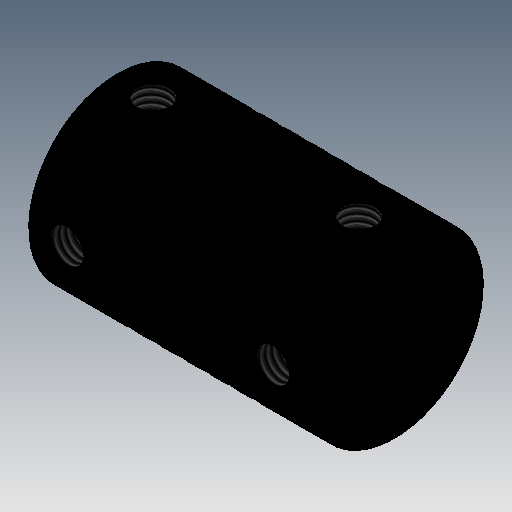
# Autodesk Inventor part: MCJN14-4-4_body
Saved by Autodesk Inventor 2019.4 (Build 234330000, 330)
## iProperties
Category: PARTsolutions
Company: MISUMI
Created: 2019-06-16
Part Number: MCJN14-4-4_body
Material: 一般
Catalog Web Link: www.cadenas.de
Description: MCJN_body-Couplings - Resin Type
Vendor: MISUMI
Document SubType Name: Modeling
Designer: psadmin
Manufacturer: MISUMI
Mass: 2.07781 g
Surface Area: 25.8504 cm^2
Volume: 2.07781 cm^3
Density: 1 g/cm^3
Appearance: PSOLRGB-0-0-0
PSOL_IDENT_0: {$CADENAS_DATA\23d-libs\misumi\metric\50_couplings\mcjn.prj},175 {VTYP=3D},{NB=MCJN14-4-4_body},{LIN
PSOL_IDENT_1: A=MCJN14-4-4},{NN=MCJN_body},{DATE=30.03.2018 07:24:16},{GEOMDATE=10.09.2008 06:56:00},{VERSION=},{L
PSOL_IDENT_2: INEID=20},{WBVAR=DD1,DD2},{WBNUMERIC=}  {NB=MCJN14-4-4_body},{LINA=MCJN14-4-4},{KT=DUMMY},{PN=MCJN14
PSOL_IDENT_3: -4-4},{MAT=Glass Fiber Reinforced PBT Resin},{AC=Set Screw},{TYPE=MCJN},{NO=14},{DD1=4},{DD1ALG1='4'
PSOL_IDENT_4: ,'4'},{DD1ALG2=4},{DD2=4},{DD2ALG1='2.5','2.5','3','3','3.2','3.2','4','4'},{DD2ALG2=4},{D=13.5},{DI
PSOL_IDENT_5: A=13.500},{L=21},{L1=21},{LL1=21},{LL11=21.000},{LL=5.3},{F=2.7},{M=M3X5},{T=0.2},{DL=4},{DR=4},{TSI
PSOL_IDENT_6: MD=3.000},{TSIMIN=2.459},{DIA1=2.8400},{L11=0.950},{L2=3.780},{L3=1.900},{TSS=3.000},{LSS=5.000}
NN: MCJN_body
NT: Couplings - Resin Type
NB: MCJN14-4-4_body
NBSYN: $TYPE.$NO.-$DD1.-$DD2._body
LINA: MCJN14-4-4
PN: MCJN14-4-4
MAT: Glass Fiber Reinforced PBT Resin
AC: Set Screw
NO: 14
DD1: 4
DD2: 4
D: 13.5
L: 21
LL: 5.3
F: 2.7
M: M3X5
T: 0.2
SUPPLIER: MISUMI
ARTICLENO: MCJN14-4-4_body
BOMINFO: MCJN14-4-4
CREATOR: CADENAS GmbH
Title: MCJN14-4-4
Author: Cadenas PARTsolutions
Comments: Couplings - Resin Type
Autodesk Inventor part; units mm, degrees
sketch "Sketch_1" plane through (0, 0, 0) normal (0, 0, 1) x (1, 0, 0)
  line L0 (21, 0) -> (0, 0)
  line L1 (0, 0) -> (0, 6.75)
  line L2 (0, 6.75) -> (21, 6.75)
  line L3 (21, 6.75) -> (21, 0)
  line L4 (21, 0) -> (0, 0)
  constraints: 10 end point
revolve "Revolution1" add sketch "Sketch_1" angle 360 about axis through (21, 0, 0) along (1, 0, 0)
sketch "Sketch_2" plane through (0, 0, 0) normal (0, 0, 1) x (1, 0, 0)
  line L0 (15.7, 0) -> (0, 0)
  line L1 (0, 0) -> (0, 2)
  line L2 (0, 2) -> (15.7, 2)
  line L3 (15.7, 2) -> (15.7, 0)
  line L4 (15.7, 0) -> (0, 0)
  constraints: 10 end point
revolve "Revolution2" cut sketch "Sketch_2" angle 360 about axis through (15.7, 0, 0) along (1, 0, 0)
sketch "Sketch3" plane through (21, 0, 0) normal (1, 0, 0) x (0, 0, -1)
  point P0 (0, 0)
hole "Hole1" at (21, 0, 0) direction (-1, 0, 0) diameter 4 depth 5.3
sketch "Sketch_4" plane through (0, 0, 0) normal (0, 0, 1) x (1, 0, 0)
  arc A0 (5.3, 1.9) -> (6.25, 1.9) centre (5.775, 1.9) ccw
  line L0 (6.25, 1.9) -> (6.25, 6.75)
  line L1 (6.25, 6.75) -> (9.125, 6.75)
  line L2 (9.125, 6.75) -> (9.125, 1.9)
  arc A1 (9.125, 1.9) -> (10.075, 1.9) centre (9.6, 1.9) ccw
  line L3 (10.075, 1.9) -> (10.075, 6.75)
  line L4 (10.075, 6.75) -> (12.85, 6.75)
  line L5 (12.85, 6.75) -> (12.85, 1.9)
  arc A2 (12.85, 1.9) -> (13.8, 1.9) centre (13.325, 1.9) ccw
  line L6 (13.8, 1.9) -> (13.8, 8.1)
  line L7 (13.8, 8.1) -> (5.3, 8.1)
  line L8 (5.3, 8.1) -> (5.3, 1.9)
  constraints: 18 end point, 6 point on circle, 3 centre point
extrude "Extrusion1" cut sketch "Sketch_4" along normal mid plane 13.5
sketch "Sketch_5" plane through (0, 0, 0) normal (0, 0, 1) x (1, 0, 0)
  line L0 (5.3, -1.9) -> (5.3, -8.1)
  line L1 (5.3, -8.1) -> (13.8, -8.1)
  line L2 (13.8, -8.1) -> (13.8, -1.9)
  arc A0 (13.8, -1.9) -> (12.85, -1.9) centre (13.325, -1.9) ccw
  line L3 (12.85, -1.9) -> (12.85, -6.75)
  line L4 (12.85, -6.75) -> (10.075, -6.75)
  line L5 (10.075, -6.75) -> (10.075, -1.9)
  arc A1 (10.075, -1.9) -> (9.125, -1.9) centre (9.6, -1.9) ccw
  line L6 (9.125, -1.9) -> (9.125, -6.75)
  line L7 (9.125, -6.75) -> (6.25, -6.75)
  line L8 (6.25, -6.75) -> (6.25, -1.9)
  arc A2 (6.25, -1.9) -> (5.3, -1.9) centre (5.775, -1.9) ccw
  constraints: 18 end point, 6 point on circle, 3 centre point
extrude "Extrusion2" cut sketch "Sketch_5" along normal mid plane 13.5
sketch "Sketch_6" plane through (0, 0, 0) normal (0, 1, 0) x (-1, 0, 0)
  arc A0 (-7.2, -1.9) -> (-8.15, -1.9) centre (-7.675, -1.9) ccw
  line L0 (-8.15, -1.9) -> (-8.15, -6.75)
  line L1 (-8.15, -6.75) -> (-11.025, -6.75)
  line L2 (-11.025, -6.75) -> (-11.025, -1.9)
  arc A1 (-11.025, -1.9) -> (-11.975, -1.9) centre (-11.5, -1.9) ccw
  line L3 (-11.975, -1.9) -> (-11.975, -6.75)
  line L4 (-11.975, -6.75) -> (-14.75, -6.75)
  line L5 (-14.75, -6.75) -> (-14.75, -1.9)
  arc A2 (-14.75, -1.9) -> (-15.7, -1.9) centre (-15.225, -1.9) ccw
  line L6 (-15.7, -1.9) -> (-15.7, -8.1)
  line L7 (-15.7, -8.1) -> (-7.2, -8.1)
  line L8 (-7.2, -8.1) -> (-7.2, -1.9)
  constraints: 18 end point, 6 point on circle, 3 centre point
extrude "Extrusion3" cut sketch "Sketch_6" along normal mid plane 13.5
sketch "Sketch_7" plane through (0, 0, 0) normal (0, 1, 0) x (-1, 0, 0)
  line L0 (-7.2, 1.9) -> (-7.2, 8.1)
  line L1 (-7.2, 8.1) -> (-15.7, 8.1)
  line L2 (-15.7, 8.1) -> (-15.7, 1.9)
  arc A0 (-15.7, 1.9) -> (-14.75, 1.9) centre (-15.225, 1.9) ccw
  line L3 (-14.75, 1.9) -> (-14.75, 6.75)
  line L4 (-14.75, 6.75) -> (-11.975, 6.75)
  line L5 (-11.975, 6.75) -> (-11.975, 1.9)
  arc A1 (-11.975, 1.9) -> (-11.025, 1.9) centre (-11.5, 1.9) ccw
  line L6 (-11.025, 1.9) -> (-11.025, 6.75)
  line L7 (-11.025, 6.75) -> (-8.15, 6.75)
  line L8 (-8.15, 6.75) -> (-8.15, 1.9)
  arc A2 (-8.15, 1.9) -> (-7.2, 1.9) centre (-7.675, 1.9) ccw
  constraints: 18 end point, 6 point on circle, 3 centre point
extrude "Extrusion4" cut sketch "Sketch_7" along normal mid plane 13.5
sketch "Sketch_8" plane through (2.7, 0, 0) normal (1, 0, 0) x (0, 0, -1)
  line L0 (0, 0) -> (0, 6.75)
  line L1 (0, 6.75) -> (1.5, 6.75)
  line L2 (1.5, 6.75) -> (1.2295, 6.4795)
  line L3 (1.2295, 6.4795) -> (1.2295, 0)
  line L4 (1.2295, 0) -> (0, 0)
  line L5 (0, 0) -> (0, 6.75)
  constraints: 12 end point
revolve "Revolution3" cut sketch "Sketch_8" angle 360 about axis through (2.7, 0, 0) along (0, -1, 0)
thread "Thread1" size "M3x0.5" class "6H" standard "ISO Metric profile" length 4.4795
sketch "Sketch_9" plane through (2.7, 0, 0) normal (1, 0, 0) x (0, 0, -1)
  line L0 (0, 0) -> (-6.75, 0)
  line L1 (-6.75, 0) -> (-6.75, 1.5)
  line L2 (-6.75, 1.5) -> (-6.4795, 1.2295)
  line L3 (-6.4795, 1.2295) -> (0, 1.2295)
  line L4 (0, 1.2295) -> (0, 0)
  line L5 (0, 0) -> (-6.75, 0)
  constraints: 12 end point
revolve "Revolution4" cut sketch "Sketch_9" angle 360 about axis through (2.7, 0, 0) along (0, 0, -1)
thread "Thread2" size "M3x0.5" class "6H" standard "ISO Metric profile" length 4.4795
sketch "Sketch_10" plane through (18.3, 0, 0) normal (1, 0, 0) x (0, 0, -1)
  line L0 (0, 0) -> (0, 6.75)
  line L1 (0, 6.75) -> (1.5, 6.75)
  line L2 (1.5, 6.75) -> (1.2295, 6.4795)
  line L3 (1.2295, 6.4795) -> (1.2295, 0)
  line L4 (1.2295, 0) -> (0, 0)
  line L5 (0, 0) -> (0, 6.75)
  constraints: 12 end point
revolve "Revolution5" cut sketch "Sketch_10" angle 360 about axis through (18.3, 0, 0) along (0, -1, 0)
thread "Thread3" size "M3x0.5" class "6H" standard "ISO Metric profile" length 4.4795
sketch "Sketch_11" plane through (18.3, 0, 0) normal (1, 0, 0) x (0, 0, -1)
  line L0 (0, 0) -> (-6.75, 0)
  line L1 (-6.75, 0) -> (-6.75, 1.5)
  line L2 (-6.75, 1.5) -> (-6.4795, 1.2295)
  line L3 (-6.4795, 1.2295) -> (0, 1.2295)
  line L4 (0, 1.2295) -> (0, 0)
  line L5 (0, 0) -> (-6.75, 0)
  constraints: 12 end point
revolve "Revolution6" cut sketch "Sketch_11" angle 360 about axis through (18.3, 0, 0) along (0, 0, -1)
thread "Thread4" size "M3x0.5" class "6H" standard "ISO Metric profile" length 4.4795
ref_plane "cp1_XY" through (2.7, 6.75, 0) normal (0, 1, 0) x (1, 0, 0)
ref_plane "cp1_YZ" through (2.7, 6.75, 0) normal (1, 0, 0) x (0, 0, -1)
ref_plane "cp1_ZX" through (2.7, 6.75, 0) normal (0, 0, -1) x (0, 1, 0)
ref_plane "cp2_XY" through (18.3, 6.75, 0) normal (0, 1, 0) x (1, 0, 0)
ref_plane "cp2_YZ" through (18.3, 6.75, 0) normal (1, 0, 0) x (0, 0, -1)
ref_plane "cp2_ZX" through (18.3, 6.75, 0) normal (0, 0, -1) x (0, 1, 0)
ref_plane "cp3_XY" through (2.7, 0, 6.75) normal (0, 0, 1) x (1, 0, 0)
ref_plane "cp3_YZ" through (2.7, 0, 6.75) normal (1, 0, 0) x (0, 1, 0)
ref_plane "cp3_ZX" through (2.7, 0, 6.75) normal (0, 1, 0) x (0, 0, 1)
ref_plane "cp4_XY" through (18.3, 0, 6.75) normal (0, 0, 1) x (1, 0, 0)
ref_plane "cp4_YZ" through (18.3, 0, 6.75) normal (1, 0, 0) x (0, 1, 0)
ref_plane "cp4_ZX" through (18.3, 0, 6.75) normal (0, 1, 0) x (0, 0, 1)
body "Solid1"
